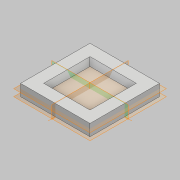
# Autodesk Inventor part: Placa - Bolsillo 50°, Profundidad 10 mm
Saved by Autodesk Inventor 2017 (Build 210142000, 142)
## iProperties
Part Number: Placa - Bolsillo 50°, Profundidad 10 mm
Material: Genérico
Document SubType Name: Modeling
Designer: franc
Density: 1 g/cm^3
Appearance: Valor por defecto
Author: franc
Autodesk Inventor part; units mm, degrees
sketch "Boceto1" plane through (0, 0, 0) normal (0, 0, 1) x (1, 0, 0)
  line L0 (-75, 75) -> (75, 75)
  line L1 (75, 75) -> (75, -75)
  line L2 (75, -75) -> (-75, -75)
  line L3 (-75, -75) -> (-75, 75)
  line L4 (-75, 75) -> (75, -75) construction
  line L5 (75, 75) -> (-75, -75) construction
  point P0 (0, 0)
  dimension "d0" = 150
  dimension "d1" = 150
  constraints: 12 end point, 2 midpoint, 2 parallel, 1 horizontal, 1 perpendicular
  measures "d0" distance of L1.end L2.end
  measures "d1" distance of L0.end L1.end
extrude "Extrusión1" add sketch "Boceto1" along normal blind 25
sketch "Boceto2" plane through (0, 0, 25) normal (0, 0, 1) x (1, 0, 0)
  line L0 (-50, 50) -> (50, 50)
  line L1 (50, 50) -> (50, -50)
  line L2 (50, -50) -> (-50, -50)
  line L3 (-50, -50) -> (-50, 50)
  line L4 (-50, 50) -> (50, -50) construction
  line L5 (50, 50) -> (-50, -50) construction
  point P0 (0, 0)
  dimension "d4" = 100
  dimension "d5" = 100
  constraints: 12 end point, 2 midpoint, 2 parallel, 1 horizontal, 1 perpendicular
  measures "d4" distance of L1.end L2.end
  measures "d5" distance of L0.end L1.end
ref_plane "Plano de trabajo1" through (0, 0, 15) normal (0, 0, 1) x (1, 0, 0)
sketch "Boceto4" plane through (0, 0, 15) normal (0, 0, 1) x (1, 0, 0)
  line L0 (-41.5714, 41.5714) -> (41.5714, 41.5714)
  line L1 (41.5714, 41.5714) -> (41.5714, -41.5714)
  line L2 (41.5714, -41.5714) -> (-41.5714, -41.5714)
  line L3 (-41.5714, -41.5714) -> (-41.5714, 41.5714)
  line L4 (-41.5714, 41.5714) -> (41.5714, -41.5714) construction
  line L5 (41.5714, 41.5714) -> (-41.5714, -41.5714) construction
  point P0 (0, 0)
  dimension "d9" = 83.1428
  dimension "d10" = 83.1428
  constraints: 12 end point, 2 midpoint, 2 parallel, 1 horizontal, 1 perpendicular
  measures "d9" distance of L1.end L2.end
  measures "d10" distance of L0.end L1.end
loft "Solevación1" cut profiles "Boceto2", "Boceto4"
